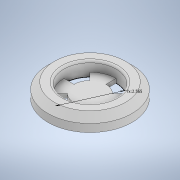
# Autodesk Inventor part: Dowel_Tube_Mount
Saved by Autodesk Inventor 2020 (Build 240168000, 168)
## iProperties
Created: 2020-03-07
Part Number: Dowel_Tube_Mount
Material: Generic
Document SubType Name: Modeling
Designer: antho
Density: 1 g/cm^3
Appearance: Default
Author: antho
Autodesk Inventor part; units mm, degrees
ref_plane "YZ Plane" through (0, 0, 0) normal (1, 0, 0) x (0, 1, 0)
ref_plane "XZ Plane" through (0, 0, 0) normal (0, 1, 0) x (-1, 0, 0)
ref_plane "XY Plane" through (0, 0, 0) normal (0, 0, 1) x (1, 0, 0)
sketch "Sketch1" plane through (0, 0, 0) normal (0, 1, 0) x (-1, 0, 0)
  circle A0 centre (0, 0) radius 12.825
  circle A1 centre (0, 0) radius 7.9375
  circle A2 centre (0, 0) radius 7.825
  circle A3 centre (0, 0) radius 20.6248
  dimension "TubeDiameter" = 25.65
  dimension "RodDiameter" = 15.875
  dimension "RodGuardDiameter" = 15.65
  dimension "HiltGuardDiameter" = 41.2496
  constraints: 4 centre point, 4 coincident
  measures "TubeDiameter" diameter of A0
  measures "RodDiameter" diameter of A1
  measures "RodGuardDiameter" diameter of A2
  measures "HiltGuardDiameter" diameter of A3
extrude "Tube&DowelMount" add sketch "Sketch1" along normal blind 5 contours A3
sketch "Sketch23" plane through (0, 0, 0) normal (0, -1, 0) x (1, 0, 0)
  circle A0 centre (0, 0) radius 20.6248
  line L0 (0, 0) -> (0, -20.6248)
  circle A1 centre (0, 0) radius 20.6248 projected
  circle A2 centre (0, 0) radius 7.825
  circle A3 centre (0, 0) radius 12.825
  line L1 (0, 0) -> (14.5839, -14.5839)
  line L2 (0, 0) -> (20.6248, 0)
  line L3 (0, 0) -> (14.5839, 14.5839)
  line L4 (0, 0) -> (0, 20.6248)
  line L5 (0, 0) -> (-14.5839, 14.5839)
  line L6 (0, 0) -> (-20.6248, 0)
  line L7 (0, 0) -> (-14.5839, -14.5839)
  point P0 (0, -12.825)
  point P1 (0, -7.825)
  point P2 (5.5331, -5.5331)
  point P3 (9.0686, -9.0686)
  point P4 (-9.0686, -9.0686)
  point P5 (-12.825, 0)
  point P6 (-7.825, 0)
  point P7 (-5.5331, -5.5331)
  point P8 (7.825, 0)
  point P9 (5.5331, 5.5331)
  point P10 (9.0686, 9.0686)
  point P11 (12.825, 0)
  point P12 (0, 7.825)
  point P13 (-5.5331, 5.5331)
  point P14 (-9.0686, 9.0686)
  point P15 (0, 12.825)
  dimension "d128" = 41.2496
  dimension "d129" = 15.65
  dimension "d130" = 25.65
  dimension "d133" = 360
  constraints: 16 end point, 3 centre point, 3 coincident, 1 vertical, 1 vertical alignment, 26 other
  measures "d128" diameter of A0
  measures "d129" diameter of A2
  measures "d130" diameter of A3
extrude "WireHole" add sketch "Sketch23" along normal blind 2 contours L2 A3 L3 A0 | A0 L1 A3 L2 | L3 A3 L4 A0 | A0 L0 A3 L1 | A3 L1 A2 L2 | L4 A3 L5 A0 | L3 A2 L4 A3 | A0 L7 A3 L0 | L2 L3 A2 | A2 L1 L2 | L5 A3 L6 A0 | L3 L4 A2 | A0 L6 A3 L7 | A3 L7 A2 L0 | A2 L0 L1 | L5 A2 L4 | L6 A2 L5 | L7 A2 L6 | L0 A2 L7 | L5 A2 L6 A3
sketch "Sketch25" plane through (0, -2, 0) normal (0, -1, 0) x (1, 0, 0)
  circle A0 centre (0, 0) radius 12.825
  dimension "d138" = 25.65
  constraints: 1 centre point, 1 coincident
  measures "d138" diameter of A0
chamfer "Chamfer4" distance 3.175 angle 45 1 edges at (20.6248, 5, 0)
fillet "Fillet2" radius 1 1 edges at (12.825, 5, 0)
equation "\"Clearance_1\" = 5"
body "Solid1"
